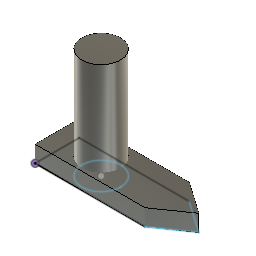
Honeycomb bed pin v2 (Autodesk Fusion 360 design; units mm, degrees)
Autodesk Fusion 360 part; units mm, degrees
sketch "Sketch1" plane through (0, 0, 0) normal (0, 0, 1) x (1, 0, 0)
  line L0 (0, 0) -> (20, 0)
  line L1 (20, 8) -> (0, 8)
  line L2 (0, 8) -> (0, 0)
  line L3 (20, 0) -> (25.7446, 4)
  line L4 (25.7446, 4) -> (20, 8)
  circle A0 centre (8, 4) radius 3.5
  dimension "d1" = 20
  dimension "d2" = 8
  dimension "d3" = 7
  dimension "d4" = 7
  dimension "d9" = 8
  constraint horizontal L0
  constraint horizontal L1
  constraint vertical L2
  constraint coincident L0.start L2.end
  measures "d1" distance of L0.start L0.end
  measures "d2" distance of L0.start L1.end
  measures "d3" distance of L0.end L3.end
  measures "d4" diameter of A0
  measures "d9" distance of L2 A0.centre
extrude "Extrude1" add sketch "Sketch1" along normal blind 3
extrude "Extrude2" add sketch "Sketch1" along normal blind 20 contours A0
named bodies: "Honeycomb bed pin"
